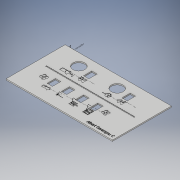
# Autodesk Inventor part: Caixa control - tapa
Saved by Autodesk Inventor 2019 (Build 230136000, 136)
## iProperties
Created: 2018-08-29
Part Number: Caixa control - tapa
Material: Genérico
Document SubType Name: Modeling
Designer: Albert Garangou Culebras
Density: 1 g/cm^3
Appearance: Valor por defecto
Author: Albert Garangou Culebras
Autodesk Inventor part; units mm, degrees
(part 1 of 2)
ref_plane "YZ Plane" through (0, 0, 0) normal (1, 0, 0) x (0, 1, 0)
ref_plane "XZ Plane" through (0, 0, 0) normal (0, 1, 0) x (-1, 0, 0)
ref_plane "XY Plane" through (0, 0, 0) normal (0, 0, 1) x (1, 0, 0)
sketch "Boceto1" plane through (0, 0, 0) normal (0, 1, 0) x (-1, 0, 0)
  line L0 (0, 0) -> (-180, 0)
  line L1 (-180, 0) -> (-180, -100)
  line L2 (-180, -100) -> (0, -100)
  line L3 (0, -100) -> (0, 0)
  dimension "d0" = 180
  dimension "d1" = 100
  constraints: 8 end point, 2 parallel, 1 horizontal, 1 perpendicular
  measures "d0" distance of L2.end L1.end
  measures "d1" distance of L1.end L0.end
extrude "base" add sketch "Boceto1" along normal blind 2
sketch "Boceto2" plane through (0, 2, 0) normal (0, 1, 0) x (1, 0, 0)
  line L0 (0, 100) -> (0, 0) projected
  line L1 (0, 0) -> (180, 0) projected
  line L2 (0, 100) -> (180, 100)
  line L3 (180, 100) -> (180, 0)
  line L4 (180, 0) -> (0, 0)
  line L5 (0, 0) -> (0, 100)
  line L6 (180, 50) -> (180, 0)
  line L7 (180, 0) -> (84.2308, 0)
  line L8 (180, 100) -> (0, 100) projected
  circle A0 centre (43.2308, 80) radius 10
  circle A1 centre (108.2308, 80) radius 10
  line L9 (61.2308, 77) -> (61.2308, 70)
  line L10 (61.2308, 70) -> (65.7308, 70)
  line L11 (65.7308, 84) -> (61.2308, 84)
  line L12 (61.2308, 84) -> (61.2308, 70)
  line L13 (65.7308, 70) -> (70.2308, 70)
  line L14 (70.2308, 70) -> (70.2308, 84)
  line L15 (70.2308, 84) -> (61.2308, 84)
  line L16 (126.2308, 70) -> (130.7308, 70)
  line L17 (126.2308, 84) -> (126.2308, 70)
  line L18 (130.7308, 70) -> (135.2308, 70)
  line L19 (135.2308, 70) -> (135.2308, 84)
  line L20 (135.2308, 84) -> (126.2308, 84)
  line L21 (61.2308, 70) -> (65.7308, 70)
  line L22 (61.2308, 84) -> (61.2308, 70)
  line L23 (65.7308, 70) -> (70.2308, 70)
  line L24 (70.2308, 70) -> (70.2308, 84)
  line L25 (70.2308, 84) -> (61.2308, 84)
  line L26 (50.4618, 35) -> (50.4618, 42)
  line L27 (50.4618, 42) -> (41.4618, 42)
  line L28 (41.4618, 42) -> (41.4618, 28)
  line L29 (41.4618, 28) -> (50.4618, 28)
  line L30 (50.4618, 28) -> (50.4618, 36)
  line L31 (65.4618, 35) -> (65.4618, 42)
  line L32 (65.4618, 42) -> (74.4618, 42)
  line L33 (74.4618, 42) -> (74.4618, 28)
  line L34 (74.4618, 28) -> (65.4618, 28)
  line L35 (65.4618, 28) -> (65.4618, 35)
  line L36 (89.4618, 35) -> (89.4618, 42)
  line L37 (89.4618, 42) -> (98.4618, 42)
  line L38 (98.4618, 42) -> (98.4618, 28)
  line L39 (98.4618, 28) -> (89.4618, 28)
  line L40 (89.4618, 28) -> (89.4618, 35)
  line L41 (113.4618, 42) -> (122.4618, 42)
  line L42 (122.4618, 42) -> (122.4618, 28)
  line L43 (122.4618, 28) -> (113.4618, 28)
  line L44 (113.4618, 28) -> (113.4618, 42)
  line L45 (84.2308, 0) -> (84.2308, 57)
  constraints: 86 end point, 15 perpendicular, 6 horizontal, 6 vertical, 4 parallel, 4 point on line, 2 centre point, 2 collinear
extrude "forats" cut sketch "Boceto2" against normal blind 26.25 contours A0 | A1 | L12 L11 L15 L14 L13 L10 L9 | L17 L20 L19 L18 L16 | L30 L29 L28 L27 L26 | L31 L32 L33 L34 L35 | L36 L37 L38 L39 L40 | L41 L42 L43 L44
sketch "Boceto3" plane through (0, 2, 0) normal (0, 1, 0) x (1, 0, 0)
  line L0 (44.524, 64.25) -> (44.524, 63.6)
  line L1 (44.5241, 59.0703) -> (44.5241, 59.7203)
  line L2 (46.4878, 61.6702) -> (46.4946, 62.3202)
  line L3 (46.4946, 62.3202) -> (47.7945, 62.3067)
  line L4 (46.4878, 61.6702) -> (46.4811, 61.0203)
  line L5 (46.4811, 61.0203) -> (47.7809, 61.0067)
  line L6 (50.3738, 61) -> (51.6738, 61) construction
  line L7 (51.6738, 61) -> (51.6738, 58.3797) construction
  spline S0 degree 2 poles (50.3738, 61) (51.6738, 61) (51.6738, 58.3797) knots 1 1 1 2 2 2
  line L8 (50.3739, 62.2797) -> (52.9738, 62.2797) construction
  line L9 (52.9738, 62.2797) -> (52.9738, 58.3797) construction
  spline S1 degree 2 poles (50.3739, 62.2797) (52.9738, 62.2797) (52.9738, 58.3797) knots 1 1 1 2 2 2
  line L10 (47.7739, 61) -> (50.3739, 61)
  line L11 (47.774, 62.3) -> (50.3739, 62.2797)
  line L12 (46.4741, 60.35) -> (44.5241, 60.3703)
  line L13 (46.5012, 62.95) -> (44.524, 62.95)
  line L14 (46.5012, 62.95) -> (46.4946, 62.3202)
  line L15 (46.4811, 61.0203) -> (46.4741, 60.35)
  line L16 (51.6738, 57.7297) -> (52.9738, 57.7297)
  line L17 (52.9738, 57.7297) -> (52.9738, 58.3797)
  line L18 (52.9738, 57.7297) -> (52.7138, 57.7297)
  line L19 (51.6738, 58.3797) -> (51.6738, 57.7297)
  line L20 (59.9327, 62.8189) -> (64.5448, 66.6583)
  line L21 (65.183, 66.3593) -> (65.183, 58.812)
  line L22 (59.9467, 62.3781) -> (64.5244, 58.5488)
  arc A0 (64.5244, 58.5488) -> (65.183, 58.812) centre (64.7675, 58.8961) ccw
  arc A1 (65.183, 66.3593) -> (64.5448, 66.6583) centre (64.7688, 66.3057) ccw
  arc A2 (59.9327, 62.8189) -> (59.9467, 62.3781) centre (60.1971, 62.6067) ccw
  line L23 (65.4041, 62.866) -> (70.0162, 66.7053)
  line L24 (70.6544, 66.4064) -> (70.6544, 58.859)
  line L25 (65.4181, 62.4251) -> (69.9959, 58.5958)
  arc A3 (69.9959, 58.5958) -> (70.6544, 58.859) centre (70.2389, 58.9431) ccw
  arc A4 (70.6544, 66.4064) -> (70.0162, 66.7053) centre (70.2402, 66.3528) ccw
  arc A5 (65.4041, 62.866) -> (65.4181, 62.4251) centre (65.6685, 62.6538) ccw
  line L26 (59.9327, 62.8189) -> (64.5448, 66.6583)
  line L27 (65.183, 66.3593) -> (65.183, 58.812)
  line L28 (59.9467, 62.3781) -> (64.5244, 58.5488)
  arc A6 (64.5244, 58.5488) -> (65.183, 58.812) centre (64.7675, 58.8961) ccw
  arc A7 (65.183, 66.3593) -> (64.5448, 66.6583) centre (64.7688, 66.3057) ccw
  arc A8 (59.9327, 62.8189) -> (59.9467, 62.3781) centre (60.1971, 62.6067) ccw
  line L29 (70.6544, 66.4064) -> (70.6544, 58.859)
  arc A9 (70.6544, 66.4064) -> (70.0162, 66.7053) centre (70.2402, 66.3528) ccw
  arc A10 (69.9959, 58.5958) -> (70.6544, 58.859) centre (70.2389, 58.9431) ccw
  line L30 (65.4041, 62.866) -> (70.0162, 66.7053)
  line L31 (65.4181, 62.4251) -> (69.9959, 58.5958)
  arc A11 (65.4041, 62.866) -> (65.4181, 62.4251) centre (65.6685, 62.6538) ccw
  line L32 (125.0045, 63.3109) -> (129.618, 67.1513)
  line L33 (130.2549, 66.8528) -> (130.2549, 59.3039)
  line L34 (125.0186, 62.87) -> (129.5963, 59.0407)
  arc A12 (129.5963, 59.0407) -> (130.2549, 59.3039) centre (129.8394, 59.3881) ccw
  arc A13 (125.0045, 63.3109) -> (125.0186, 62.87) centre (125.2689, 63.0987) ccw
  line L35 (135.7263, 66.8984) -> (135.7263, 59.351)
  arc A14 (135.0677, 59.0878) -> (135.7263, 59.351) centre (135.3108, 59.4351) ccw
  line L36 (130.4759, 63.358) -> (135.0881, 67.1973)
  line L37 (130.49, 62.9171) -> (135.0677, 59.0878)
  arc A15 (130.4759, 63.358) -> (130.49, 62.9171) centre (130.7404, 63.1457) ccw
  arc A16 (130.2549, 66.8528) -> (129.618, 67.1513) centre (129.8665, 66.8528) ccw
  arc A17 (135.7263, 66.8984) -> (135.0881, 67.1973) centre (135.3283, 66.8795) ccw
  arc A18 (106.6796, 62.0746) -> (106.6915, 62.6002) centre (110.6758, 62.2469) ccw
  spline S2 degree 3 poles (106.6915, 62.6002) (105.0998, 62.0414) (103.5694, 61.7201) (101.554, 61.7539) knots 0 0 0 0 1 1 1 1
  circle A19 centre (110.6758, 62.2469) radius 1
  arc A20 (113.6718, 62.4018) -> (111.2741, 65.1866) centre (110.6758, 62.2469) ccw
  line L38 (113.7945, 62.0483) -> (113.441, 62.4018)
  line L39 (113.7945, 62.0483) -> (114.1481, 62.4018)
  arc A21 (113.9221, 62.4018) -> (111.2741, 65.4413) centre (110.6758, 62.2469) ccw
  line L40 (114.1481, 62.4018) -> (113.9221, 62.4018)
  line L41 (113.6718, 62.4018) -> (113.441, 62.4018)
  line L42 (107.6078, 62.9219) -> (105.7752, 62.2785) construction
  arc A22 (105.9542, 62.3567) -> (107.4193, 62.871) centre (99.7742, 82.3035) ccw construction
  line L43 (101.554, 61.7539) -> (101.5559, 61.261)
  line L44 (111.2741, 65.4413) -> (111.2741, 65.1866)
  line L45 (44.524, 64.25) -> (44.524, 64.38)
  line L46 (44.524, 64.25) -> (44.524, 65.55)
  line L47 (44.524, 65.55) -> (42.574, 65.55)
  line L48 (42.574, 65.55) -> (42.574, 64.25)
  line L49 (42.574, 64.25) -> (31.524, 64.25)
  line L50 (31.524, 59.05) -> (31.524, 64.25)
  line L51 (42.574, 59.05) -> (42.574, 57.75)
  line L52 (42.574, 57.75) -> (44.5239, 57.75)
  line L53 (44.5241, 57.75) -> (44.5241, 59.0703)
  line L54 (42.574, 59.05) -> (31.524, 59.05)
  line L55 (51.2122, 23.1412) -> (51.2122, 22.6162)
  line L56 (51.2122, 18.9576) -> (51.2122, 19.4826)
  line L57 (52.7873, 20.0076) -> (51.2122, 20.0076)
  line L58 (52.7872, 22.0912) -> (51.2122, 22.0912)
  line L59 (52.7872, 22.0912) -> (52.7872, 21.599)
  line L60 (52.7873, 20.549) -> (52.7873, 20.0076)
  line L61 (51.2122, 23.1412) -> (51.2122, 23.2462)
  line L62 (51.2122, 23.1412) -> (51.2122, 24.1912)
  line L63 (51.2122, 24.1912) -> (49.6372, 24.1912)
  line L64 (49.6372, 24.1912) -> (49.6372, 23.1412)
  line L65 (49.6372, 23.1412) -> (40.7122, 23.1412)
  line L66 (40.7122, 18.9412) -> (40.7122, 23.1412)
  line L67 (49.6372, 18.9412) -> (49.6372, 17.8912)
  line L68 (49.6372, 17.8912) -> (51.2122, 17.8912)
  line L69 (51.2122, 17.8912) -> (51.2122, 18.9576)
  line L70 (49.6372, 18.9412) -> (40.7122, 18.9412)
  line L71 (51.2122, 20.0076) -> (51.2122, 19.4826)
  line L72 (51.2122, 22.0912) -> (51.2122, 22.6162)
  line L73 (44.5241, 60.3703) -> (44.5241, 59.7203)
  line L74 (44.524, 63.6) -> (44.524, 62.95)
  line L75 (52.7872, 21.374) -> (52.4873, 21.374)
  line L76 (52.4873, 21.374) -> (52.4873, 20.774)
  line L77 (52.4873, 20.774) -> (52.7873, 20.774)
  line L78 (52.7873, 20.774) -> (52.7873, 20.549)
  line L79 (52.7872, 21.599) -> (52.7872, 21.374)
  line L80 (89.627, 23.9855) -> (97.277, 23.9855)
  line L81 (97.277, 16.3355) -> (89.627, 16.3355)
  line L82 (89.627, 16.3355) -> (89.627, 23.9855)
  line L83 (67.3452, 22.5781) -> (66.2952, 22.5781)
  line L84 (66.2952, 22.5781) -> (66.2952, 21.8781)
  line L85 (67.3452, 21.8781) -> (67.3452, 22.5781)
  line L86 (67.3452, 21.8781) -> (67.3452, 21.9481)
  line L87 (67.3452, 21.8781) -> (67.3452, 21.5281)
  line L88 (68.3953, 21.1781) -> (67.3452, 21.1781)
  line L89 (68.3953, 19.7765) -> (67.3452, 19.7781)
  line L90 (67.3452, 19.0781) -> (67.3452, 19.4281)
  line L91 (67.3452, 18.3671) -> (67.3452, 19.0781)
  line L92 (66.2952, 19.0767) -> (66.2952, 18.3767)
  line L93 (66.2952, 18.3767) -> (67.3452, 18.3767)
  line L94 (68.3953, 20.1375) -> (68.3953, 19.7765)
  line L95 (67.3452, 19.7781) -> (67.3452, 19.4281)
  line L96 (67.3452, 21.1781) -> (67.3452, 21.5281)
  line L97 (68.3953, 20.2875) -> (68.3953, 20.1375)
  line L98 (68.3953, 21.1781) -> (68.3953, 20.7896)
  line L99 (65.2366, 21.8767) -> (65.2366, 19.0767)
  line L100 (65.2366, 21.8781) -> (66.2952, 21.8781)
  line L101 (65.2366, 19.0767) -> (66.2952, 19.0767)
  line L102 (97.277, 23.9855) -> (97.277, 20.798)
  line L103 (97.277, 19.523) -> (97.277, 16.3355)
  line L104 (100.5679, 20.798) -> (100.5679, 19.523)
  line L105 (100.5679, 19.523) -> (97.277, 19.523)
  line L106 (97.277, 20.798) -> (100.5679, 20.798)
  line L107 (122.2298, 31.1299) -> (122.2298, 16.1299)
  line L108 (122.2298, 16.1299) -> (113.2298, 16.1299)
  line L109 (113.2298, 26.1299) -> (113.2298, 21.1299)
  line L110 (113.2298, 26.1299) -> (113.2298, 25.6299)
  line L111 (113.2298, 21.1299) -> (113.2298, 21.6299)
  line L112 (113.2298, 21.6299) -> (113.2298, 20.6299)
  line L113 (113.2298, 16.1299) -> (114.2298, 16.1299)
  line L114 (122.2298, 16.1299) -> (121.2298, 16.1299)
  line L115 (113.2298, 16.1299) -> (113.2298, 17.1299)
  line L116 (114.2298, 25.6299) -> (121.2298, 25.6299)
  line L117 (121.2298, 25.6299) -> (121.2298, 21.6299)
  line L118 (121.2298, 21.6299) -> (114.2298, 21.6299)
  line L119 (114.2298, 21.6299) -> (114.2298, 25.6299)
  line L120 (114.2298, 20.6299) -> (121.2298, 20.6299)
  line L121 (121.2298, 20.6299) -> (121.2298, 17.1299)
  line L122 (121.2298, 17.1299) -> (114.2298, 17.1299)
  line L123 (114.2298, 17.1299) -> (114.2298, 20.6299)
  line L124 (114.2298, 17.1299) -> (116.5298, 17.1299)
  line L125 (116.5298, 17.1299) -> (118.8298, 17.1299)
  line L126 (117.6798, 17.1299) -> (118.7948, 17.1299)
  line L127 (118.7948, 17.1299) -> (119.9098, 17.1299)
  line L128 (119.9098, 17.1299) -> (121.0248, 17.1299)
  circle A23 centre (120.4673, 19.4799) radius 0.45
  circle A24 centre (118.8673, 19.4799) radius 0.45
  circle A25 centre (117.2673, 19.4799) radius 0.45
  circle A26 centre (118.8673, 24.2799) radius 0.45
  circle A27 centre (120.4673, 24.2799) radius 0.45
  circle A28 centre (117.2673, 24.2799) radius 0.45
  circle A29 centre (118.8673, 29.0799) radius 0.45
  circle A30 centre (120.4673, 29.0799) radius 0.45
  circle A31 centre (117.2673, 29.0799) radius 0.45
  line L129 (114.2298, 17.1299) -> (114.2298, 18.1299)
  line L130 (114.2298, 17.1299) -> (114.9798, 17.1299)
  line L131 (114.9823, 17.6299) -> (117.0198, 17.6299)
  line L132 (117.0198, 17.6299) -> (117.0198, 18.1299)
  line L133 (117.0198, 18.1299) -> (114.9823, 18.1299)
  line L134 (114.9823, 18.1299) -> (114.9823, 17.6299)
  line L135 (114.9823, 22.6299) -> (114.9823, 22.1299)
  line L136 (114.9823, 22.1299) -> (117.0198, 22.1299)
  line L137 (117.0198, 22.6299) -> (114.9823, 22.6299)
  line L138 (117.0198, 22.1299) -> (117.0198, 22.6299)
  line L139 (114.9823, 27.6299) -> (114.9823, 27.1299)
  line L140 (117.0198, 27.6299) -> (114.9823, 27.6299)
  line L141 (117.0198, 27.1299) -> (117.0198, 27.6299)
  line L142 (114.9823, 27.1299) -> (117.0198, 27.1299)
  line L143 (121.2298, 30.6299) -> (121.2298, 26.6299)
  line L144 (40.7122, 23.1412) -> (40.7122, 18.9412)
  line L145 (49.6372, 18.9412) -> (40.7122, 18.9412)
  line L146 (49.6372, 18.9412) -> (49.6372, 17.8912)
  line L147 (49.6372, 17.8912) -> (51.2122, 17.8912)
  line L148 (51.2122, 17.8912) -> (51.2122, 20.0076)
  line L149 (51.2122, 20.0076) -> (52.7873, 20.0076)
  line L150 (52.7873, 20.0076) -> (52.7873, 20.774)
  line L151 (52.7873, 20.774) -> (52.4873, 20.774)
  line L152 (52.4873, 20.774) -> (52.4873, 21.3799)
  line L153 (52.4873, 21.3799) -> (52.7872, 21.3799)
  line L154 (52.7872, 21.3799) -> (52.7872, 22.0908)
  line L155 (52.7872, 22.0908) -> (51.2122, 22.0908)
  line L156 (51.2122, 22.0908) -> (51.2122, 24.1912)
  line L157 (49.6372, 24.1912) -> (51.2122, 24.1912)
  line L158 (49.6372, 24.1912) -> (49.6372, 23.1412)
  line L159 (49.6372, 23.1412) -> (40.7122, 23.1412)
  line L160 (40.7122, 23.1412) -> (40.7122, 18.9412)
  line L161 (31.524, 64.25) -> (31.524, 59.05)
  line L162 (31.524, 59.05) -> (42.574, 59.05)
  line L163 (42.574, 57.75) -> (42.574, 59.05)
  line L164 (42.574, 57.75) -> (44.5241, 57.75)
  line L165 (44.5241, 57.75) -> (44.5241, 60.3703)
  line L166 (44.5241, 60.3703) -> (46.4741, 60.35)
  line L167 (46.4741, 60.35) -> (46.4811, 61.0203)
  line L168 (46.4811, 61.0203) -> (46.5012, 62.95)
  line L169 (46.5012, 62.95) -> (44.524, 62.95)
  line L170 (44.524, 62.95) -> (44.524, 65.55)
  line L171 (44.524, 65.55) -> (42.574, 65.55)
  line L172 (42.574, 65.55) -> (42.574, 64.25)
  line L173 (42.574, 64.25) -> (31.524, 64.25)
  line L174 (31.524, 64.25) -> (31.524, 59.05)
  line L175 (51.6738, 57.7297) -> (52.9738, 57.7297)
  line L176 (52.9738, 58.3797) -> (52.9738, 57.7297)
  line L177 (51.6738, 58.3797) -> (51.6738, 57.7297)
  line L178 (50.3739, 61) -> (51.6738, 61) construction
  line L179 (51.6738, 61) -> (51.6738, 58.3797) construction
  spline S3 degree 2 poles (50.3739, 61) (51.6738, 61) (51.6738, 58.3797) knots 1 1 1 2 2 2
  line L180 (50.3739, 62.2797) -> (52.9738, 62.2797) construction
  line L181 (52.9738, 62.2797) -> (52.9738, 58.3797) construction
  spline S4 degree 2 poles (50.3739, 62.2797) (52.9738, 62.2797) (52.9738, 58.3797) knots 1 1 1 2 2 2
  line L182 (65.2366, 21.8781) -> (65.2366, 19.0767)
  line L183 (66.2952, 19.0767) -> (65.2366, 19.0767)
  line L184 (66.2952, 19.0767) -> (66.2952, 18.3767)
  line L185 (66.2952, 18.3767) -> (67.3452, 18.3767)
  line L186 (67.3452, 18.3767) -> (67.3452, 19.7781)
  line L187 (67.3452, 19.7781) -> (68.3953, 19.7765)
  line L188 (68.3953, 20.2875) -> (68.3953, 19.7765)
  line L189 (68.3953, 20.7896) -> (68.3953, 21.1781)
  line L190 (68.3953, 21.1781) -> (67.3452, 21.1781)
  line L191 (67.3452, 21.1781) -> (67.3452, 22.5781)
  line L192 (67.3452, 22.5781) -> (66.2952, 22.5781)
  line L193 (66.2952, 22.5781) -> (66.2952, 21.8781)
  line L194 (66.2952, 21.8781) -> (65.2366, 21.8781)
  line L195 (65.2366, 21.8781) -> (65.2366, 19.0767)
  spline S5 degree 3 poles (68.3953, 20.7896) (70.7309, 20.7896) (70.1186, 19.8311) (75.3334, 20.4858) knots 0 0 0 0 1 1 1 1
  line L196 (75.3833, 20.0889) -> (75.3334, 20.4858)
  line L197 (91.5068, 17.6299) -> (92.143, 17.6299)
  line L198 (92.143, 17.6299) -> (92.143, 22.0105)
  line L199 (92.143, 22.0105) -> (93.452, 19.0299)
  line L200 (93.452, 19.0299) -> (93.8546, 19.0299)
  line L201 (93.8546, 19.0299) -> (95.1799, 22.0105)
  line L202 (95.1799, 22.0105) -> (95.1799, 17.6299)
  line L203 (95.1799, 17.6299) -> (95.8762, 17.6299)
  line L204 (95.8762, 17.6299) -> (95.8762, 22.7264)
  line L205 (94.9375, 22.7264) -> (93.6941, 19.9299)
  line L206 (93.6941, 19.9299) -> (92.4659, 22.7264)
  line L207 (91.5068, 22.7264) -> (92.4659, 22.7264)
  line L208 (91.5068, 22.7264) -> (91.5068, 17.6299)
  line L209 (94.9375, 22.7264) -> (95.8762, 22.7264)
  line L210 (113.2298, 20.6299) -> (113.2298, 17.1299)
  line L211 (114.2298, 26.6299) -> (113.2298, 26.6299)
  line L212 (113.2298, 26.6299) -> (113.2298, 26.1299)
  line L213 (114.2298, 26.6299) -> (122.2298, 26.6299)
  line L214 (46.4811, 61.0203) -> (46.4946, 62.3202)
  line L215 (68.3953, 20.7896) -> (68.3953, 20.3896)
  line L216 (68.3953, 20.3896) -> (68.3953, 19.7765)
  spline S6 degree 5 poles (106.6795, 62.0746) (105.6922, 61.7381) (104.6834, 61.4633) (103.6429, 61.3009) (102.599, 61.2445) (101.5559, 61.261) knots 0 0 0 0 0 0 1 1 1 1 1 1
  spline S7 degree 5 poles (68.3953, 20.3896) (68.7146, 20.3892) (69.033, 20.3748) (69.3533, 20.3369) (70.0068, 20.1742) (70.6554, 19.9929) (71.0064, 19.933) (72.092, 19.816) (73.1869, 19.8628) (73.9196, 19.919) (74.6528, 19.9973) (75.3833, 20.0889) knots 0 0 0 0 0 0 0.226406 0.226406 0.226406 0.477676 0.477676 0.477676 1 1 1 1 1 1
  point P0 (0, 0)
  point P1 (126.2308, 70)
  point P2 (69.8531, 20.6214)
  point P3 (70.839, 20.3816)
  point P4 (117.6798, 19.4799)
  point P5 (117.6798, 24.2799)
  point P6 (117.6798, 29.0799)
  dimension "d288" = 0.4
  dimension "d259" = 1.6
  dimension "d266" = 4.8
  dimension "d276" = 4.5
  dimension "d283" = 5
  dimension "d289" = 1
  constraints: 418 end point, 43 point on circle, 42 vertical, 36 collinear, 34 perpendicular, 32 centre point, 20 point on line, 12 horizontal, 11 parallel, 5 coincident, 3 midpoint, 1 tangent, 64 other
  measures "d259" distance of A23.centre A24.centre
  measures "d266" distance of A25.centre A28.centre
  measures "d276" distance of L131.start L135.end
  measures "d283" distance of L135.start L139.start
  measures "d289" distance of L116.start L211.start
extrude "Extrusión3" cut sketch "Boceto3" against normal blind 0.5 contours L0 L74 L13 L14 L2 L4 L15 L12 L73 L1 L53 L52 L51 L54 L50 L49 L48 L47 L46 L45 | L20 A1 L21 A0 L22 A2 | L23 A4 L24 A3 L25 A5 | L32 A16 L33 A12 L34 A13 | L35 A14 L37 A15 L36 A17 | S6 L43 S2 A18 | L55 L72 L58 L59 L79 L153 L152 L76 L77 L78 L60 L57 L71 L56 L69 L68 L67 L70 L66 L65 L64 L63 L62 L61 | L80 L102 L106 L104 L105 L103 L81 L82 | L85 L87 L96 L88 L98 L215 L216 L97 L94 L89 L95 L90 L91 L93 L92 L101 L99 L100 L84 L83 | S5 L196 S7 L215 | L107 L108 L115 L210 L112 L109 L212 L211 L213 | A23 | A24 | A25 | A26 | A27 | A28 | L134 L133 L132 L131 | L137 L138 L136 L135
sketch "Boceto5" plane through (0, 2, 0) normal (0, 1, 0) x (1, 0, 0)
  line L0 (46.5012, 62.95) -> (46.4741, 60.35) projected
  line L1 (46.4946, 62.3175) -> (46.4811, 61.0256)
  line L2 (50.4732, 62.3175) -> (46.4946, 62.3175)
  line L3 (50.4732, 62.3175) -> (52.9585, 62.3175) construction
  line L4 (52.9585, 62.3175) -> (52.9585, 58.4509) construction
  spline S0 degree 2 poles (50.4732, 62.3175) (52.9585, 62.3175) (52.9585, 58.4509) knots 1 1 1 2 2 2
  line L5 (50.4732, 61.0256) -> (51.7159, 61.0256) construction
  line L6 (51.7159, 61.0256) -> (51.7159, 58.4509) construction
  spline S1 degree 2 poles (50.4732, 61.0256) (51.7159, 61.0256) (51.7159, 58.4509) knots 1 1 1 2 2 2
  line L7 (51.7159, 58.4509) -> (52.9585, 58.4509)
  line L8 (46.4811, 61.0256) -> (50.4732, 61.0256)
  point P0 (0, 0)
  constraints: 8 end point, 3 horizontal, 2 point on line, 2 vertical, 6 other
extrude "Extrusión4" cut sketch "Boceto5" against normal blind 0.5
sketch "Boceto6" plane through (0, 2, 0) normal (0, 1, 0) x (1, 0, 0)
  spline S0 degree 4 poles (29.0799, 35.9708) (29.157, 35.7147) (29.5973, 35.6307) (29.6514, 35.9754) (29.6224, 36.5115) (30.003, 37.3994) (30.9963, 38.6611) (31.8038, 39.1799) (34.1243, 38.5401) (34.4092, 36.16) knots 0 0 0 0 0 0.168165 0.246229 0.343173 0.454491 0.580711 1 1 1 1 1
  spline S1 degree 4 poles (34.4092, 36.16) (34.7426, 35.3106) (32.7275, 33.2427) (32.5523, 36.2152) (30.5175, 34.9657) knots 0 0 0 0 0 1 1 1 1 1
  spline S2 degree 3 poles (30.5175, 34.9657) (30.1475, 33.8706) (31.9148, 35.589) (33.3235, 32.8129) knots 0 0 0 0 1 1 1 1
  spline S3 degree 4 poles (29.2384, 33.5854) (28.9714, 32.8219) (29.1741, 27.8697) (22.2623, 31.4954) (24.9254, 34.4527) knots 0 0 0 0 0 1 1 1 1 1
  spline S4 degree 3 poles (24.9254, 34.4527) (25.3025, 34.7606) (26.1651, 34.7965) (26.8468, 34.2785) knots 0 0 0 0 1 1 1 1
  spline S5 degree 3 poles (28.1827, 34.9339) (27.2948, 35.0506) (26.5081, 35.3521) (25.9075, 36.0652) knots 0 0 0 0 1 1 1 1
  spline S6 degree 3 poles (29.2384, 38.9749) (29.7153, 38.8274) (29.0086, 37.0279) (28.8371, 37.2609) knots 0 0 0 0 1 1 1 1
  spline S7 degree 2 poles (28.9441, 37.2803) (28.8496, 36.3277) (29.0799, 35.9708) knots 0 0 0 1 1 1
  spline S8 degree 4 poles (25.9075, 36.0652) (25.5031, 36.2597) (25.0891, 37.4783) (25.8436, 39.2046) (28.4119, 40.2659) (29.5743, 39.0581) (29.3681, 38.316) knots 0 0 0 0 0 0.388251 0.566915 1 1 1 1 1
  spline S9 degree 2 poles (28.1827, 34.9339) (28.2241, 34.93) (28.2695, 34.9084) knots 0 0 0 1 1 1
  line L0 (28.247, 34.9191) -> (28.2921, 34.8978) construction
  arc A0 (28.2873, 34.8994) -> (28.2513, 34.9165) centre (28.117, 34.5869) ccw construction
  spline S10 degree 4 poles (26.8468, 34.2785) (26.8742, 34.2176) (27.9219, 34.0143) (28.7341, 34.5531) (28.2695, 34.9084) knots 0 0 0 0 0 1 1 1 1 1
  line L1 (29.5064, 33.6433) -> (30.5358, 34.5853)
  line L2 (30.5358, 34.5853) -> (29.4747, 35.7449)
  line L3 (28.2695, 34.4831) -> (29.4747, 35.7449)
  line L4 (28.349, 34.5722) -> (29.2384, 33.5854)
  spline S11 degree 3 poles (29.2384, 33.5854) (29.4655, 33.9093) (30.0577, 33.5756) (30.0053, 32.599) knots 0 0 0 0 1 1 1 1
  spline S12 degree 4 poles (30.0053, 32.599) (29.9904, 32.3205) (29.8007, 31.7908) (29.1962, 30.9163) (29.973, 30.0496) (30.9102, 29.5496) (31.4961, 29.9491) (33.4717, 30.4348) (33.5063, 32.1817) knots 0 0 0 0 0 0.268483 0.383339 0.491913 0.605909 1 1 1 1 1
  spline S13 degree 2 poles (33.5063, 32.1817) (33.5448, 32.5564) (33.3235, 32.8129) knots 0 0 0 1 1 1
  point P0 (0, 0)
  point P1 (29.3679, 35.7325)
  point P2 (29.5571, 35.8001)
  point P3 (29.6292, 36.0072)
  point P4 (29.6563, 36.381)
  point P5 (29.9672, 37.2278)
  point P6 (30.607, 38.1197)
  point P7 (31.2874, 38.6375)
  point P8 (32.4634, 38.7049)
  point P9 (34.1759, 35.2829)
  point P10 (33.3695, 34.7967)
  point P11 (32.3652, 35.0292)
  point P12 (31.0767, 34.531)
  point P13 (28.9715, 32.4514)
  point P14 (27.7551, 30.9492)
  point P15 (25.3437, 31.3253)
  point P16 (25.3271, 34.6378)
  point P17 (25.9996, 34.6497)
  point P18 (27.3265, 35.1223)
  point P19 (26.5793, 35.473)
  point P20 (28.9488, 36.3448)
  point P21 (25.4858, 36.6469)
  point P22 (25.4513, 37.779)
  point P23 (26.1739, 38.9118)
  point P24 (27.6829, 39.6637)
  point P25 (29.0091, 39.3067)
  point P26 (26.9393, 34.2428)
  point P27 (27.6806, 34.2429)
  point P28 (29.4501, 33.7051)
  point P29 (29.7418, 33.5646)
  point P30 (29.9059, 32.1623)
  point P31 (29.6292, 31.4538)
  point P32 (29.5571, 30.7017)
  point P33 (30.0211, 30.0807)
  point P34 (30.5358, 29.8089)
  point P35 (31.0074, 29.7895)
  point P36 (32.0167, 30.1098)
  point P37 (33.4771, 32.5359)
  constraints: 10 end point, 2 midpoint, 1 centre point, 1 perpendicular, 1 point on circle, 73 other
sketch "Boceto8" plane through (0, 2, 0) normal (0, 1, 0) x (1, 0, 0)
  spline S0 degree 4 poles (133.7635, 35.9708) (133.8407, 35.7147) (134.281, 35.6307) (134.3351, 35.9754) (134.306, 36.5115) (134.6867, 37.3994) (135.6799, 38.6611) (136.4874, 39.1799) (138.808, 38.5401) (139.0929, 36.16) knots 0 0 0 0 0 0.168165 0.246229 0.343173 0.454491 0.580711 1 1 1 1 1
  spline S1 degree 4 poles (139.0929, 36.16) (139.4262, 35.3106) (137.4112, 33.2428) (137.2359, 36.2152) (135.2011, 34.9657) knots 0 0 0 0 0 1 1 1 1 1
  spline S2 degree 3 poles (135.2011, 34.9657) (134.8312, 33.8706) (136.5984, 35.589) (138.0072, 32.8129) knots 0 0 0 0 1 1 1 1
  spline S3 degree 4 poles (134.6889, 32.599) (134.6741, 32.3205) (134.4844, 31.7908) (133.8799, 30.9163) (134.6567, 30.0496) (135.5938, 29.5497) (136.1798, 29.9491) (138.1553, 30.4347) (138.19, 32.1817) knots 0 0 0 0 0 0.268482 0.383337 0.491911 0.605908 1 1 1 1 1
  spline S4 degree 2 poles (138.19, 32.1817) (138.2282, 32.5567) (138.0072, 32.8129) knots 0 0 0 1 1 1
  spline S5 degree 3 poles (133.9221, 33.5854) (134.1396, 33.9242) (134.7371, 33.5794) (134.6889, 32.599) knots 0 0 0 0 1 1 1 1
  line L0 (134.19, 33.6433) -> (135.2195, 34.5853)
  line L1 (135.2195, 34.5853) -> (134.1584, 35.7449)
  spline S6 degree 2 poles (132.8663, 34.9339) (132.9078, 34.93) (132.9532, 34.9084) knots 0 0 0 1 1 1
  line L2 (132.9307, 34.9191) -> (132.9757, 34.8978) construction
  arc A0 (132.971, 34.8994) -> (132.935, 34.9165) centre (132.8007, 34.5869) ccw construction
  line L3 (132.9532, 34.4831) -> (134.1584, 35.7449)
  spline S7 degree 4 poles (133.9221, 33.5854) (133.6547, 32.8228) (133.8603, 27.8652) (126.9425, 31.5019) (129.6091, 34.4527) knots 0 0 0 0 0 1 1 1 1 1
  spline S8 degree 4 poles (131.5305, 34.2785) (131.5578, 34.2176) (132.6056, 34.0143) (133.4177, 34.5531) (132.9532, 34.9084) knots 0 0 0 0 0 1 1 1 1 1
  line L4 (133.0326, 34.5722) -> (133.9221, 33.5854)
  spline S9 degree 3 poles (129.6091, 34.4527) (129.9861, 34.7608) (130.8488, 34.7963) (131.5305, 34.2785) knots 0 0 0 0 1 1 1 1
  spline S10 degree 3 poles (132.8663, 34.9339) (131.9785, 35.0506) (131.1917, 35.3522) (130.5912, 36.0652) knots 0 0 0 0 1 1 1 1
  spline S11 degree 3 poles (133.9221, 38.9749) (134.3989, 38.8274) (133.6923, 37.0279) (133.5207, 37.2609) knots 0 0 0 0 1 1 1 1
  spline S12 degree 2 poles (133.6277, 37.2803) (133.5378, 36.3241) (133.7635, 35.9708) knots 0 0 0 1 1 1
  spline S13 degree 4 poles (130.5912, 36.0652) (130.1868, 36.2596) (129.7732, 37.478) (130.5279, 39.2038) (133.0957, 40.2652) (134.2581, 39.0581) (134.0518, 38.316) knots 0 0 0 0 0 0.388242 0.566914 1 1 1 1 1
  spline S14 degree 4 poles (29.0799, 35.9708) (29.157, 35.7147) (29.5973, 35.6307) (29.6514, 35.9754) (29.6224, 36.5115) (30.003, 37.3994) (30.9963, 38.6611) (31.8038, 39.1799) (34.1243, 38.5401) (34.4092, 36.16) knots 0 0 0 0 0 0.168165 0.246229 0.343173 0.454491 0.580711 1 1 1 1 1
  spline S15 degree 4 poles (34.4092, 36.16) (34.7426, 35.3106) (32.7275, 33.2427) (32.5523, 36.2152) (30.5175, 34.9657) knots 0 0 0 0 0 1 1 1 1 1
  spline S16 degree 3 poles (30.5175, 34.9657) (30.1475, 33.8706) (31.9148, 35.589) (33.3235, 32.8129) knots 0 0 0 0 1 1 1 1
  spline S17 degree 4 poles (29.2384, 33.5854) (28.9713, 32.8221) (29.1748, 27.8685) (22.2614, 31.4971) (24.9254, 34.4527) knots 0 0 0 0 0 1 1 1 1 1
  spline S18 degree 3 poles (24.9254, 34.4527) (25.3025, 34.7607) (26.1651, 34.7965) (26.8468, 34.2785) knots 0 0 0 0 1 1 1 1
  spline S19 degree 3 poles (28.1827, 34.9339) (27.2948, 35.0506) (26.5081, 35.3521) (25.9075, 36.0652) knots 0 0 0 0 1 1 1 1
  spline S20 degree 3 poles (29.2384, 38.9749) (29.7153, 38.8274) (29.0086, 37.0279) (28.8371, 37.2609) knots 0 0 0 0 1 1 1 1
  spline S21 degree 2 poles (28.9441, 37.2803) (28.8507, 36.3268) (29.0799, 35.9708) knots 0 0 0 1 1 1
  spline S22 degree 4 poles (25.9075, 36.0652) (25.5031, 36.2597) (25.0892, 37.4783) (25.8438, 39.2044) (28.412, 40.2657) (29.5744, 39.0581) (29.3681, 38.316) knots 0 0 0 0 0 0.388249 0.566915 1 1 1 1 1
  spline S23 degree 2 poles (28.1827, 34.9339) (28.2241, 34.93) (28.2695, 34.9084) knots 0 0 0 1 1 1
  line L5 (28.247, 34.9191) -> (28.2921, 34.8978) construction
  arc A1 (28.2873, 34.8994) -> (28.2513, 34.9165) centre (28.117, 34.5869) ccw construction
  spline S24 degree 4 poles (26.8468, 34.2785) (26.8742, 34.2176) (27.9219, 34.0143) (28.7341, 34.5531) (28.2695, 34.9084) knots 0 0 0 0 0 1 1 1 1 1
  line L6 (29.5064, 33.6433) -> (30.5358, 34.5853)
  line L7 (30.5358, 34.5853) -> (29.4747, 35.7449)
  line L8 (28.2695, 34.4831) -> (29.4747, 35.7449)
  line L9 (28.349, 34.5722) -> (29.2384, 33.5854)
  spline S25 degree 3 poles (29.2384, 33.5854) (29.463, 33.9132) (30.0565, 33.5766) (30.0053, 32.599) knots 0 0 0 0 1 1 1 1
  spline S26 degree 4 poles (30.0053, 32.599) (29.9904, 32.3205) (29.8007, 31.7908) (29.1962, 30.9163) (29.973, 30.0496) (30.9102, 29.5496) (31.4961, 29.9491) (33.4717, 30.4348) (33.5063, 32.1817) knots 0 0 0 0 0 0.268483 0.383338 0.491912 0.605909 1 1 1 1 1
  spline S27 degree 2 poles (33.5063, 32.1817) (33.5447, 32.5565) (33.3235, 32.8129) knots 0 0 0 1 1 1
  point P0 (0, 0)
  point P1 (134.0516, 35.7325)
  point P2 (134.2407, 35.8001)
  point P3 (134.3129, 36.0072)
  point P4 (134.34, 36.381)
  point P5 (134.6509, 37.2278)
  point P6 (135.2907, 38.1197)
  point P7 (135.9711, 38.6375)
  point P8 (137.147, 38.7049)
  point P9 (138.8596, 35.2829)
  point P10 (138.0532, 34.7967)
  point P11 (137.0489, 35.0292)
  point P12 (135.7604, 34.531)
  point P13 (134.5896, 32.1623)
  point P14 (134.3129, 31.4539)
  point P15 (134.2407, 30.7018)
  point P16 (134.7047, 30.0807)
  point P17 (135.2195, 29.809)
  point P18 (135.691, 29.7895)
  point P19 (136.7003, 30.1098)
  point P20 (138.1607, 32.5362)
  point P21 (133.6553, 32.4513)
  point P22 (134.418, 33.5739)
  point P23 (134.1284, 33.7118)
  point P24 (132.4389, 30.949)
  point P25 (132.3643, 34.2429)
  point P26 (130.0255, 31.3276)
  point P27 (131.623, 34.2428)
  point P28 (132.0102, 35.1223)
  point P29 (130.0107, 34.6379)
  point P30 (130.6833, 34.6497)
  point P31 (131.2629, 35.4731)
  point P32 (133.635, 36.3408)
  point P33 (130.1697, 36.6466)
  point P34 (133.693, 39.3064)
  point P35 (130.1354, 37.7785)
  point P36 (132.3669, 39.6631)
  point P37 (130.858, 38.9112)
  point P38 (29.3679, 35.7325)
  point P39 (29.5571, 35.8001)
  point P40 (29.6292, 36.0072)
  point P41 (29.6563, 36.381)
  point P42 (29.9672, 37.2278)
  point P43 (30.607, 38.1197)
  point P44 (31.2874, 38.6375)
  point P45 (32.4634, 38.7049)
  point P46 (34.1759, 35.2829)
  point P47 (33.3695, 34.7967)
  point P48 (32.3652, 35.0292)
  point P49 (31.0767, 34.531)
  point P50 (28.9716, 32.4514)
  point P51 (27.7552, 30.9491)
  point P52 (25.3432, 31.3259)
  point P53 (25.3271, 34.6378)
  point P54 (25.9996, 34.6497)
  point P55 (27.3265, 35.1223)
  point P56 (26.5793, 35.473)
  point P57 (28.9494, 36.3439)
  point P58 (25.4859, 36.6468)
  point P59 (25.4514, 37.7789)
  point P60 (26.174, 38.9117)
  point P61 (27.683, 39.6635)
  point P62 (29.0092, 39.3066)
  point P63 (26.9393, 34.2428)
  point P64 (27.6806, 34.2429)
  point P65 (29.4487, 33.7069)
  point P66 (29.7398, 33.5671)
  point P67 (29.9059, 32.1623)
  point P68 (29.6292, 31.4538)
  point P69 (29.5571, 30.7018)
  point P70 (30.0211, 30.0807)
  point P71 (30.5358, 29.8089)
  point P72 (31.0074, 29.7895)
  point P73 (32.0167, 30.1098)
  point P74 (33.4771, 32.536)
  constraints: 20 end point, 4 midpoint, 2 centre point, 2 perpendicular, 2 point on circle, 146 other
extrude "Extrusión6" cut sketch "Boceto8" against normal blind 0.5 contours S0 L3 L4 S8 S6 S10 S13 S11 S12 | S0 S1 S2 L1 | L1 S2 L0 S5 L4 L3 | L4 S7 S9 S8 L3 | S11 S13 | S2 S4 S3 S5 L0 picked at (134.0684, 38.4186)
extrude "Extrusión7" cut sketch "Boceto6" against normal blind 0.5 contours S0 L3 L4 S10 S9 S5 S8 S6 S7 | S0 S1 S2 L2 | L2 S2 L1 S11 L4 L3 | L2 S2 | L4 S3 S4 S10 L3 | S2 S13 S12 S11 L1
sketch "Boceto10" plane through (0, 2, 0) normal (0, 1, 0) x (1, 0, 0)
  line L0 (131.2163, 8.6831) -> (176.264, 8.6831) construction
  line L1 (176.264, 8.6831) -> (176.264, -0.0046) construction
  line L2 (176.264, -0.0046) -> (131.2163, -0.0046) construction
  line L3 (131.2163, -0.0046) -> (131.2163, 8.6831) construction
  line L4 (131.1904, 4.5048) -> (132.5388, 8.5048)
  line L5 (132.5388, 8.5048) -> (133.1936, 8.5048)
  line L6 (133.1936, 8.5048) -> (134.5421, 4.5048)
  line L7 (134.5421, 4.5048) -> (133.9813, 4.5048)
  line L8 (133.9813, 4.5048) -> (133.6182, 5.6232)
  line L9 (133.6182, 5.6232) -> (132.0915, 5.6232)
  line L10 (132.0915, 5.6232) -> (131.7284, 4.5048)
  line L11 (131.7284, 4.5048) -> (131.1904, 4.5048)
  line L12 (133.4724, 6.077) -> (132.8532, 7.9603)
  line L13 (132.8532, 7.9603) -> (132.2374, 6.077)
  line L14 (132.2374, 6.077) -> (133.4724, 6.077)
  line L15 (135.3978, 4.5048) -> (134.8921, 4.5048)
  line L16 (134.8921, 4.5048) -> (134.8921, 8.6831)
  line L17 (134.8921, 8.6831) -> (135.3978, 8.6831)
  line L18 (135.3978, 8.6831) -> (135.3978, 4.5048)
  spline S0 degree 2 poles (138.6555, 6.0543) (138.6555, 5.3185) (137.9424, 4.4206) (137.4043, 4.4206) knots 0 0 0 1 2 2 2
  spline S1 degree 2 poles (137.4043, 4.4206) (137.1612, 4.4206) (136.8143, 4.5405) (136.6458, 4.6442) knots 0 0 0 1 2 2 2
  line L19 (136.6458, 4.6442) -> (136.6134, 4.5048)
  line L20 (136.6134, 4.5048) -> (136.1401, 4.5048)
  line L21 (136.1401, 4.5048) -> (136.1401, 8.6831)
  line L22 (136.1401, 8.6831) -> (136.6458, 8.6831)
  line L23 (136.6458, 8.6831) -> (136.6458, 7.192)
  spline S2 degree 2 poles (136.6458, 7.192) (136.837, 7.3638) (137.2811, 7.5907) (137.5631, 7.5907) knots 0 0 0 1 2 2 2
  spline S3 degree 2 poles (137.5631, 7.5907) (138.072, 7.5907) (138.6555, 6.7771) (138.6555, 6.0543) knots 0 0 0 1 2 2 2
  spline S4 degree 2 poles (138.1336, 6.0154) (138.1336, 6.5535) (137.8062, 7.111) (137.4432, 7.111) knots 0 0 0 1 2 2 2
  spline S5 degree 2 poles (137.4432, 7.111) (137.239, 7.111) (136.8176, 6.9165) (136.6458, 6.7674) knots 0 0 0 1 2 2 2
  line L24 (136.6458, 6.7674) -> (136.6458, 5.0462)
  spline S6 degree 2 poles (136.6458, 5.0462) (136.837, 4.9522) (137.132, 4.8744) (137.307, 4.8744) knots 0 0 0 1 2 2 2
  spline S7 degree 2 poles (137.307, 4.8744) (137.6928, 4.8744) (138.1336, 5.4222) (138.1336, 6.0154) knots 0 0 0 1 2 2 2
  spline S8 degree 2 poles (140.4837, 4.4368) (139.7641, 4.4368) (138.9732, 5.2439) (138.9732, 5.9894) knots 0 0 0 1 2 2 2
  spline S9 degree 2 poles (138.9732, 5.9894) (138.9732, 6.722) (139.7414, 7.5907) (140.3605, 7.5907) knots 0 0 0 1 2 2 2
  spline S10 degree 2 poles (140.3605, 7.5907) (140.6393, 7.5907) (141.0704, 7.4287) (141.2293, 7.2569) knots 0 0 0 1 2 2 2
  spline S11 degree 2 poles (141.2293, 7.2569) (141.3913, 7.0851) (141.5631, 6.5891) (141.5631, 6.2293) knots 0 0 0 1 2 2 2
  line L25 (141.5631, 6.2293) -> (141.5631, 5.9538)
  line L26 (141.5631, 5.9538) -> (139.4853, 5.9538)
  spline S12 degree 2 poles (139.4853, 5.9538) (139.4853, 5.4319) (140.0105, 4.8776) (140.4772, 4.8776) knots 0 0 0 1 2 2 2
  spline S13 degree 2 poles (140.4772, 4.8776) (140.6425, 4.8776) (140.9635, 4.9522) (141.0931, 5.0105) knots 0 0 0 1 2 2 2
  spline S14 degree 2 poles (141.0931, 5.0105) (141.2293, 5.0753) (141.4173, 5.1888) (141.4788, 5.2407) knots 0 0 0 1 2 2 2
  line L27 (141.4788, 5.2407) -> (141.508, 5.2407)
  line L28 (141.508, 5.2407) -> (141.508, 4.6896)
  spline S15 degree 2 poles (141.508, 4.6896) (141.4205, 4.654) (141.1547, 4.5502) (141.051, 4.521) knots 0 0 0 1 2 2 2
  spline S16 degree 2 poles (141.051, 4.521) (140.9051, 4.4789) (140.6652, 4.4368) (140.4837, 4.4368) knots 0 0 0 1 2 2 2
  spline S17 degree 2 poles (141.0704, 6.3395) (141.0639, 6.5437) (140.9797, 6.842) (140.8986, 6.9424) knots 0 0 0 1 2 2 2
  spline S18 degree 2 poles (140.8986, 6.9424) (140.8111, 7.0559) (140.5356, 7.1758) (140.3314, 7.1758) knots 0 0 0 1 2 2 2
  spline S19 degree 2 poles (140.3314, 7.1758) (140.1304, 7.1758) (139.8484, 7.0559) (139.7317, 6.9392) knots 0 0 0 1 2 2 2
  spline S20 degree 2 poles (139.7317, 6.9392) (139.6182, 6.8193) (139.5015, 6.5308) (139.4853, 6.3395) knots 0 0 0 1 2 2 2
  line L29 (139.4853, 6.3395) -> (141.0704, 6.3395)
  line L30 (143.6669, 6.9651) -> (143.6409, 6.9651)
  spline S21 degree 2 poles (143.6409, 6.9651) (143.5826, 6.9813) (143.4562, 6.9878) (143.3686, 6.9878) knots 0 0 0 1 2 2 2
  spline S22 degree 2 poles (143.3686, 6.9878) (143.1644, 6.9878) (142.7625, 6.8095) (142.581, 6.6345) knots 0 0 0 1 2 2 2
  line L31 (142.581, 6.6345) -> (142.581, 4.5048)
  line L32 (142.581, 4.5048) -> (142.0753, 4.5048)
  line L33 (142.0753, 4.5048) -> (142.0753, 7.5065)
  line L34 (142.0753, 7.5065) -> (142.581, 7.5065)
  line L35 (142.581, 7.5065) -> (142.581, 7.0591)
  spline S23 degree 2 poles (142.581, 7.0591) (142.8565, 7.3055) (143.2682, 7.5065) (143.4626, 7.5065) knots 0 0 0 1 2 2 2
  spline S24 degree 2 poles (143.4626, 7.5065) (143.5404, 7.5065) (143.6182, 7.5) (143.6669, 7.4903) knots 0 0 0 1 2 2 2
  line L36 (143.6669, 7.4903) -> (143.6669, 6.9651)
  spline S25 degree 2 poles (144.9667, 4.4465) (144.555, 4.4465) (144.0915, 4.9165) (144.0915, 5.4254) knots 0 0 0 1 2 2 2
  line L37 (144.0915, 5.4254) -> (144.0915, 7.0883)
  line L38 (144.0915, 7.0883) -> (143.7511, 7.0883)
  line L39 (143.7511, 7.0883) -> (143.7511, 7.5065)
  line L40 (143.7511, 7.5065) -> (144.0915, 7.5065)
  line L41 (144.0915, 7.5065) -> (144.0915, 8.3687)
  line L42 (144.0915, 8.3687) -> (144.5972, 8.3687)
  line L43 (144.5972, 8.3687) -> (144.5972, 7.5065)
  line L44 (144.5972, 7.5065) -> (145.5275, 7.5065)
  line L45 (145.5275, 7.5065) -> (145.5275, 7.0883)
  line L46 (145.5275, 7.0883) -> (144.5972, 7.0883)
  line L47 (144.5972, 7.0883) -> (144.5972, 5.6588)
  spline S26 degree 2 poles (144.5972, 5.6588) (144.5972, 5.4319) (144.6134, 5.1823) (144.6685, 5.0753) knots 0 0 0 1 2 2 2
  spline S27 degree 2 poles (144.6685, 5.0753) (144.7139, 4.9813) (144.9181, 4.8873) (145.0931, 4.8873) knots 0 0 0 1 2 2 2
  spline S28 degree 2 poles (145.0931, 4.8873) (145.2163, 4.8873) (145.4464, 4.9619) (145.4983, 4.9846) knots 0 0 0 1 2 2 2
  line L48 (145.4983, 4.9846) -> (145.5275, 4.9846)
  line L49 (145.5275, 4.9846) -> (145.5275, 4.5308)
  spline S29 degree 2 poles (145.5275, 4.5308) (145.3848, 4.4919) (145.0931, 4.4465) (144.9667, 4.4465) knots 0 0 0 1 2 2 2
  spline S30 degree 2 poles (149.333, 4.427) (148.9083, 4.427) (148.2049, 4.6864) (147.9521, 4.9489) knots 0 0 0 1 2 2 2
  spline S31 degree 2 poles (147.9521, 4.9489) (147.6993, 5.2147) (147.4302, 5.9992) (147.4302, 6.5081) knots 0 0 0 1 2 2 2
  spline S32 degree 2 poles (147.4302, 6.5081) (147.4302, 6.9911) (147.7025, 7.7561) (147.9553, 8.0283) knots 0 0 0 1 2 2 2
  spline S33 degree 2 poles (147.9553, 8.0283) (148.1985, 8.2909) (148.9116, 8.5762) (149.3362, 8.5762) knots 0 0 0 1 2 2 2
  spline S34 degree 2 poles (149.3362, 8.5762) (149.5404, 8.5762) (149.91, 8.5178) (150.0785, 8.4659) knots 0 0 0 1 2 2 2
  spline S35 degree 2 poles (150.0785, 8.4659) (150.2147, 8.427) (150.5453, 8.2844) (150.6458, 8.2326) knots 0 0 0 1 2 2 2
  line L50 (150.6458, 8.2326) -> (150.6458, 7.5907)
  line L51 (150.6458, 7.5907) -> (150.6004, 7.5907)
  spline S36 degree 2 poles (150.6004, 7.5907) (150.4999, 7.6783) (150.2892, 7.8371) (150.0947, 7.9279) knots 0 0 0 1 2 2 2
  spline S37 degree 2 poles (150.0947, 7.9279) (149.9327, 8.0089) (149.5145, 8.1159) (149.2746, 8.1159) knots 0 0 0 1 2 2 2
  spline S38 degree 2 poles (149.2746, 8.1159) (148.6976, 8.1159) (147.9845, 7.2471) (147.9845, 6.5243) knots 0 0 0 1 2 2 2
  spline S39 degree 2 poles (147.9845, 6.5243) (147.9845, 6.1223) (148.1725, 5.5194) (148.3508, 5.312) knots 0 0 0 1 2 2 2
  spline S40 degree 2 poles (148.3508, 5.312) (148.5226, 5.1045) (149.0088, 4.8873) (149.3135, 4.8873) knots 0 0 0 1 2 2 2
  spline S41 degree 2 poles (149.3135, 4.8873) (149.5372, 4.8873) (149.9845, 4.9522) (150.1369, 5.017) knots 0 0 0 1 2 2 2
  line L52 (150.1369, 5.017) -> (150.1369, 6.051)
  line L53 (150.1369, 6.051) -> (149.2098, 6.051)
  line L54 (149.2098, 6.051) -> (149.2098, 6.5178)
  line L55 (149.2098, 6.5178) -> (150.662, 6.5178)
  line L56 (150.662, 6.5178) -> (150.662, 4.7706)
  spline S42 degree 2 poles (150.662, 4.7706) (150.5615, 4.7253) (150.2179, 4.5859) (150.072, 4.5437) knots 0 0 0 1 2 2 2
  spline S43 degree 2 poles (150.072, 4.5437) (149.8743, 4.4854) (149.5566, 4.427) (149.333, 4.427) knots 0 0 0 1 2 2 2
  spline S44 degree 2 poles (152.9635, 4.8225) (152.9019, 4.7771) (152.6944, 4.6151) (152.5972, 4.5664) knots 0 0 0 1 2 2 2
  spline S45 degree 2 poles (152.5972, 4.5664) (152.4643, 4.4951) (152.2147, 4.4206) (151.9878, 4.4206) knots 0 0 0 1 2 2 2
  spline S46 degree 2 poles (151.9878, 4.4206) (151.803, 4.4206) (151.4691, 4.5599) (151.3427, 4.6864) knots 0 0 0 1 2 2 2
  spline S47 degree 2 poles (151.3427, 4.6864) (151.2228, 4.8095) (151.0769, 5.1726) (151.0769, 5.3736) knots 0 0 0 1 2 2 2
  spline S48 degree 2 poles (151.0769, 5.3736) (151.0769, 5.6847) (151.3395, 6.1256) (151.6247, 6.252) knots 0 0 0 1 2 2 2
  spline S49 degree 2 poles (151.6247, 6.252) (151.8776, 6.3687) (152.5647, 6.4562) (152.9635, 6.4789) knots 0 0 0 1 2 2 2
  line L57 (152.9635, 6.4789) -> (152.9635, 6.5762)
  spline S50 degree 2 poles (152.9635, 6.5762) (152.9635, 6.7512) (152.8565, 6.9684) (152.7592, 7.03) knots 0 0 0 1 2 2 2
  spline S51 degree 2 poles (152.7592, 7.03) (152.662, 7.0916) (152.3832, 7.1304) (152.2341, 7.1304) knots 0 0 0 1 2 2 2
  spline S52 degree 2 poles (152.2341, 7.1304) (152.0591, 7.1304) (151.5858, 7.0267) (151.3492, 6.9262) knots 0 0 0 1 2 2 2
  line L58 (151.3492, 6.9262) -> (151.32, 6.9262)
  line L59 (151.32, 6.9262) -> (151.32, 7.4416)
  spline S53 degree 2 poles (151.32, 7.4416) (151.4594, 7.4805) (151.9813, 7.5778) (152.2374, 7.5778) knots 0 0 0 1 2 2 2
  spline S54 degree 2 poles (152.2374, 7.5778) (152.5485, 7.5778) (152.9732, 7.4805) (153.1417, 7.3541) knots 0 0 0 1 2 2 2
  spline S55 degree 2 poles (153.1417, 7.3541) (153.307, 7.2309) (153.4691, 6.8387) (153.4691, 6.5567) knots 0 0 0 1 2 2 2
  line L60 (153.4691, 6.5567) -> (153.4691, 4.5048)
  line L61 (153.4691, 4.5048) -> (152.9635, 4.5048)
  line L62 (152.9635, 4.5048) -> (152.9635, 4.8225)
  line L63 (152.9635, 5.2439) -> (152.9635, 6.077)
  spline S56 degree 2 poles (152.9635, 6.077) (152.7819, 6.0608) (152.2341, 6.0057) (152.0623, 5.9538) knots 0 0 0 1 2 2 2
  spline S57 degree 2 poles (152.0623, 5.9538) (151.8613, 5.8922) (151.5988, 5.6361) (151.5988, 5.4092) knots 0 0 0 1 2 2 2
  spline S58 degree 2 poles (151.5988, 5.4092) (151.5988, 5.1499) (151.8905, 4.8873) (152.1693, 4.8873) knots 0 0 0 1 2 2 2
  spline S59 degree 2 poles (152.1693, 4.8873) (152.4059, 4.8873) (152.7949, 5.0916) (152.9635, 5.2439) knots 0 0 0 1 2 2 2
  line L64 (155.7706, 6.9651) -> (155.7447, 6.9651)
  spline S60 degree 2 poles (155.7447, 6.9651) (155.6863, 6.9813) (155.5599, 6.9878) (155.4724, 6.9878) knots 0 0 0 1 2 2 2
  spline S61 degree 2 poles (155.4724, 6.9878) (155.2682, 6.9878) (154.8662, 6.8095) (154.6847, 6.6345) knots 0 0 0 1 2 2 2
  line L65 (154.6847, 6.6345) -> (154.6847, 4.5048)
  line L66 (154.6847, 4.5048) -> (154.179, 4.5048)
  line L67 (154.179, 4.5048) -> (154.179, 7.5065)
  line L68 (154.179, 7.5065) -> (154.6847, 7.5065)
  line L69 (154.6847, 7.5065) -> (154.6847, 7.0591)
  spline S62 degree 2 poles (154.6847, 7.0591) (154.9602, 7.3055) (155.3719, 7.5065) (155.5664, 7.5065) knots 0 0 0 1 2 2 2
  spline S63 degree 2 poles (155.5664, 7.5065) (155.6442, 7.5065) (155.722, 7.5) (155.7706, 7.4903) knots 0 0 0 1 2 2 2
  line L70 (155.7706, 7.4903) -> (155.7706, 6.9651)
  spline S64 degree 2 poles (157.8354, 4.8225) (157.7738, 4.7771) (157.5664, 4.6151) (157.4691, 4.5664) knots 0 0 0 1 2 2 2
  spline S65 degree 2 poles (157.4691, 4.5664) (157.3362, 4.4951) (157.0866, 4.4206) (156.8597, 4.4206) knots 0 0 0 1 2 2 2
  spline S66 degree 2 poles (156.8597, 4.4206) (156.675, 4.4206) (156.3411, 4.5599) (156.2147, 4.6864) knots 0 0 0 1 2 2 2
  spline S67 degree 2 poles (156.2147, 4.6864) (156.0947, 4.8095) (155.9489, 5.1726) (155.9489, 5.3736) knots 0 0 0 1 2 2 2
  spline S68 degree 2 poles (155.9489, 5.3736) (155.9489, 5.6847) (156.2114, 6.1256) (156.4967, 6.252) knots 0 0 0 1 2 2 2
  spline S69 degree 2 poles (156.4967, 6.252) (156.7495, 6.3687) (157.4367, 6.4562) (157.8354, 6.4789) knots 0 0 0 1 2 2 2
  line L71 (157.8354, 6.4789) -> (157.8354, 6.5762)
  spline S70 degree 2 poles (157.8354, 6.5762) (157.8354, 6.7512) (157.7284, 6.9684) (157.6312, 7.03) knots 0 0 0 1 2 2 2
  spline S71 degree 2 poles (157.6312, 7.03) (157.534, 7.0916) (157.2552, 7.1304) (157.1061, 7.1304) knots 0 0 0 1 2 2 2
  spline S72 degree 2 poles (157.1061, 7.1304) (156.931, 7.1304) (156.4578, 7.0267) (156.2211, 6.9262) knots 0 0 0 1 2 2 2
  line L72 (156.2211, 6.9262) -> (156.192, 6.9262)
  line L73 (156.192, 6.9262) -> (156.192, 7.4416)
  spline S73 degree 2 poles (156.192, 7.4416) (156.3314, 7.4805) (156.8532, 7.5778) (157.1093, 7.5778) knots 0 0 0 1 2 2 2
  spline S74 degree 2 poles (157.1093, 7.5778) (157.4205, 7.5778) (157.8451, 7.4805) (158.0137, 7.3541) knots 0 0 0 1 2 2 2
  spline S75 degree 2 poles (158.0137, 7.3541) (158.179, 7.2309) (158.3411, 6.8387) (158.3411, 6.5567) knots 0 0 0 1 2 2 2
  line L74 (158.3411, 6.5567) -> (158.3411, 4.5048)
  line L75 (158.3411, 4.5048) -> (157.8354, 4.5048)
  line L76 (157.8354, 4.5048) -> (157.8354, 4.8225)
  line L77 (157.8354, 5.2439) -> (157.8354, 6.077)
  spline S76 degree 2 poles (157.8354, 6.077) (157.6539, 6.0608) (157.1061, 6.0057) (156.9343, 5.9538) knots 0 0 0 1 2 2 2
  spline S77 degree 2 poles (156.9343, 5.9538) (156.7333, 5.8922) (156.4707, 5.6361) (156.4707, 5.4092) knots 0 0 0 1 2 2 2
  spline S78 degree 2 poles (156.4707, 5.4092) (156.4707, 5.1499) (156.7625, 4.8873) (157.0412, 4.8873) knots 0 0 0 1 2 2 2
  spline S79 degree 2 poles (157.0412, 4.8873) (157.2779, 4.8873) (157.6669, 5.0916) (157.8354, 5.2439) knots 0 0 0 1 2 2 2
  line L78 (161.4075, 4.5048) -> (160.9019, 4.5048)
  line L79 (160.9019, 4.5048) -> (160.9019, 6.2163)
  spline S80 degree 2 poles (160.9019, 6.2163) (160.9019, 6.4238) (160.863, 6.7804) (160.8046, 6.8873) knots 0 0 0 1 2 2 2
  spline S81 degree 2 poles (160.8046, 6.8873) (160.743, 7.0008) (160.5226, 7.111) (160.3346, 7.111) knots 0 0 0 1 2 2 2
  spline S82 degree 2 poles (160.3346, 7.111) (160.1466, 7.111) (159.7479, 6.91) (159.5566, 6.748) knots 0 0 0 1 2 2 2
  line L80 (159.5566, 6.748) -> (159.5566, 4.5048)
  line L81 (159.5566, 4.5048) -> (159.051, 4.5048)
  line L82 (159.051, 4.5048) -> (159.051, 7.5065)
  line L83 (159.051, 7.5065) -> (159.5566, 7.5065)
  line L84 (159.5566, 7.5065) -> (159.5566, 7.1726)
  spline S83 degree 2 poles (159.5566, 7.1726) (159.7835, 7.3768) (160.2212, 7.5907) (160.4675, 7.5907) knots 0 0 0 1 2 2 2
  spline S84 degree 2 poles (160.4675, 7.5907) (160.9083, 7.5907) (161.4075, 7.0073) (161.4075, 6.453) knots 0 0 0 1 2 2 2
  line L85 (161.4075, 6.453) -> (161.4075, 4.5048)
  spline S85 degree 2 poles (162.2244, 4.0251) (162.2763, 4.0024) (162.474, 3.9311) (162.6004, 3.9019) knots 0 0 0 1 2 2 2
  spline S86 degree 2 poles (162.6004, 3.9019) (162.7398, 3.8663) (162.9764, 3.8241) (163.1158, 3.8241) knots 0 0 0 1 2 2 2
  spline S87 degree 2 poles (163.1158, 3.8241) (163.3492, 3.8241) (163.6733, 3.9473) (163.7641, 4.0575) knots 0 0 0 1 2 2 2
  spline S88 degree 2 poles (163.7641, 4.0575) (163.8516, 4.1677) (163.9197, 4.4562) (163.9197, 4.641) knots 0 0 0 1 2 2 2
  line L86 (163.9197, 4.641) -> (163.9197, 4.9035)
  spline S89 degree 2 poles (163.9197, 4.9035) (163.7155, 4.7253) (163.3233, 4.5567) (163.0283, 4.5567) knots 0 0 0 1 2 2 2
  spline S90 degree 2 poles (163.0283, 4.5567) (162.5161, 4.5567) (161.91, 5.3185) (161.91, 6.0348) knots 0 0 0 1 2 2 2
  spline S91 degree 2 poles (161.91, 6.0348) (161.91, 6.4076) (162.1207, 6.9846) (162.2957, 7.1888) knots 0 0 0 1 2 2 2
  spline S92 degree 2 poles (162.2957, 7.1888) (162.4643, 7.38) (162.9278, 7.5907) (163.1741, 7.5907) knots 0 0 0 1 2 2 2
  spline S93 degree 2 poles (163.1741, 7.5907) (163.4075, 7.5907) (163.7479, 7.4805) (163.9197, 7.38) knots 0 0 0 1 2 2 2
  line L87 (163.9197, 7.38) -> (163.9489, 7.5065)
  line L88 (163.9489, 7.5065) -> (164.4254, 7.5065)
  line L89 (164.4254, 7.5065) -> (164.4254, 4.8484)
  spline S94 degree 2 poles (164.4254, 4.8484) (164.4254, 4.0834) (163.7609, 3.3703) (163.0769, 3.3703) knots 0 0 0 1 2 2 2
  spline S95 degree 2 poles (163.0769, 3.3703) (162.8565, 3.3703) (162.3962, 3.4416) (162.1985, 3.5) knots 0 0 0 1 2 2 2
  line L90 (162.1985, 3.5) -> (162.1985, 4.0251)
  line L91 (162.1985, 4.0251) -> (162.2244, 4.0251)
  line L92 (163.9197, 5.3185) -> (163.9197, 6.9684)
  spline S96 degree 2 poles (163.9197, 6.9684) (163.7317, 7.0591) (163.414, 7.1369) (163.2552, 7.1369) knots 0 0 0 1 2 2 2
  spline S97 degree 2 poles (163.2552, 7.1369) (162.8727, 7.1369) (162.4318, 6.5729) (162.4318, 6.0446) knots 0 0 0 1 2 2 2
  spline S98 degree 2 poles (162.4318, 6.0446) (162.4318, 5.5454) (162.7657, 5.0235) (163.1417, 5.0235) knots 0 0 0 1 2 2 2
  spline S99 degree 2 poles (163.1417, 5.0235) (163.3395, 5.0235) (163.7544, 5.1791) (163.9197, 5.3185) knots 0 0 0 1 2 2 2
  spline S100 degree 2 poles (167.6247, 6.0057) (167.6247, 5.2471) (166.8954, 4.4206) (166.286, 4.4206) knots 0 0 0 1 2 2 2
  spline S101 degree 2 poles (166.286, 4.4206) (165.6604, 4.4206) (164.944, 5.2731) (164.944, 6.0057) knots 0 0 0 1 2 2 2